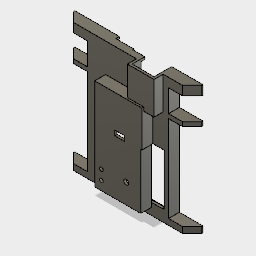
lpcCNC_Lid v15 (Autodesk Fusion 360 design; units mm, degrees)
Autodesk Fusion 360 part; units mm, degrees
sketch "Base Sketch" plane through (0, 0, 0) normal (0, 0, 1) x (1, 0, 0)
  line L0 (0, 0) -> (106, 0)
  line L1 (106, 0) -> (106, 106)
  line L2 (106, 106) -> (0, 106)
  line L3 (0, 106) -> (0, 0)
  line L4 (19.5, 106) -> (86.5, 106)
  line L5 (86.5, 106) -> (86.5, 0)
  line L6 (86.5, 0) -> (19.5, 0)
  line L7 (19.5, 0) -> (19.5, 106)
  line L8 (21.5, 3) -> (84.5, 3)
  line L9 (84.5, 3) -> (84.5, 104)
  line L10 (84.5, 104) -> (21.5, 104)
  line L11 (21.5, 104) -> (21.5, 3)
  circle A0 centre (23, 7) radius 3
  circle A1 centre (23, 7) radius 0.9
  circle A2 centre (83, 7) radius 0.9
  circle A3 centre (83, 7) radius 3
  circle A4 centre (83, 99) radius 0.9
  circle A5 centre (83, 99) radius 3
  circle A6 centre (23, 99) radius 0.9
  circle A7 centre (23, 99) radius 3
  line L12 (80, 106) -> (80, 104)
  line L13 (52, 106) -> (52, 104)
  line L14 (37, 106) -> (37, 104)
  line L15 (86.5, 5) -> (106, 5)
  line L16 (106, 5) -> (106, 0)
  line L17 (106, 0) -> (86.5, 0)
  line L18 (86.5, 0) -> (86.5, 5)
  line L19 (0, 5) -> (19.5, 5)
  line L20 (19.5, 5) -> (19.5, 0)
  line L21 (19.5, 0) -> (0, 0)
  line L22 (0, 0) -> (0, 5)
  line L23 (86.5, 106) -> (106, 106)
  line L24 (106, 106) -> (106, 98.5)
  line L25 (106, 98.5) -> (86.5, 98.5)
  line L26 (86.5, 98.5) -> (86.5, 106)
  line L27 (0, 106) -> (19.5, 106)
  line L28 (19.5, 106) -> (19.5, 98.5)
  line L29 (19.5, 98.5) -> (0, 98.5)
  line L30 (0, 98.5) -> (0, 106)
  line L31 (106, 76.5) -> (86.5, 76.5)
  line L32 (86.5, 76.5) -> (86.5, 80)
  line L33 (86.5, 80) -> (106, 80)
  line L34 (106, 80) -> (106, 76.5)
  line L35 (0, 76.5) -> (19.5, 76.5)
  line L36 (19.5, 76.5) -> (19.5, 80)
  line L37 (19.5, 80) -> (0, 80)
  line L38 (0, 80) -> (0, 76.5)
  line L39 (63.5, 104) -> (80, 104)
  line L40 (80, 104) -> (80, 81)
  line L41 (36.5, 8) -> (71.5, 8)
  line L42 (71.5, 52) -> (83, 52)
  line L43 (83, 52) -> (83, 9.5)
  line L44 (83, 9.5) -> (71.5, 9.5)
  line L45 (71.5, 9.5) -> (71.5, 52)
  line L46 (62, 106) -> (62, 104)
  line L47 (62, 104) -> (62, 81)
  line L48 (36.5, 80) -> (71.5, 80)
  line L49 (36.5, 80) -> (36.5, 8)
  line L50 (71.5, 8) -> (71.5, 80)
  line L51 (62, 81) -> (80, 81)
  line L52 (36.5, 80) -> (62, 80)
  line L53 (62, 80) -> (62, 82)
  line L54 (62, 82) -> (36.5, 82)
  line L55 (36.5, 82) -> (36.5, 80)
  line L56 (62, 106) -> (60, 106)
  line L57 (60, 106) -> (60, 82)
  line L58 (60, 82) -> (62, 82)
  line L59 (62, 82) -> (62, 106)
  line L60 (80, 81) -> (82, 81)
  line L61 (82, 81) -> (82, 106)
  line L62 (82, 106) -> (80, 106)
  line L63 (80, 106) -> (80, 81)
  line L64 (82, 81) -> (71.5, 81)
  line L65 (71.5, 81) -> (71.5, 79)
  line L66 (71.5, 79) -> (82, 79)
  line L67 (82, 79) -> (82, 81)
  line L68 (71.5, 79) -> (73.5, 79)
  line L69 (73.5, 79) -> (73.5, 52)
  line L70 (73.5, 52) -> (71.5, 52)
  line L71 (71.5, 52) -> (71.5, 79)
  line L72 (36.5, 82) -> (34.5, 82)
  line L73 (34.5, 82) -> (34.5, 6)
  line L74 (34.5, 6) -> (36.5, 6)
  line L75 (36.5, 6) -> (36.5, 82)
  line L76 (36.5, 6) -> (71.5, 6)
  line L77 (71.5, 6) -> (71.5, 8)
  line L78 (71.5, 8) -> (36.5, 8)
  line L79 (36.5, 8) -> (36.5, 6)
  line L80 (71.5, 6) -> (72.5, 6)
  line L81 (72.5, 6) -> (72.5, 52)
  line L82 (72.5, 52) -> (71.5, 52)
  line L83 (71.5, 52) -> (71.5, 6)
  line L84 (62, 81) -> (73.5, 81)
  line L85 (73.5, 81) -> (73.5, 82)
  line L86 (73.5, 82) -> (62, 82)
  line L87 (62, 82) -> (62, 81)
  line L88 (73.5, 81) -> (73.5, 79)
  line L89 (51, 55) -> (59, 55)
  line L90 (59, 55) -> (59, 51)
  line L91 (59, 51) -> (51, 51)
  line L92 (51, 51) -> (51, 55)
  circle A8 centre (60.5, 22.5) radius 2
  circle A9 centre (40, 21.5) radius 1.5
  circle A10 centre (40, 13.5) radius 1.5
  dimension "d1" = 106
  dimension "d2" = 106
  dimension "d4" = 67
  dimension "d5" = 19.5
  dimension "d6" = 63
  dimension "d8" = 2
  dimension "d9" = 3
  dimension "d10" = 6
  dimension "d12" = 6
  dimension "d13" = 6
  dimension "d14" = 6
  dimension "d15" = 23
  dimension "d16" = 23
  dimension "d17" = 23
  dimension "d18" = 23
  dimension "d19" = 7
  dimension "d20" = 7
  dimension "d21" = 7
  dimension "d22" = 7
  dimension "d24" = 2
  dimension "d25" = 6.5
  dimension "d28" = 15
  dimension "d35" = 5
  dimension "d36" = 5
  dimension "d37" = 7.5
  dimension "d38" = 7.5
  dimension "d39" = 3.5
  dimension "d40" = 26
  dimension "d41" = 3.5
  dimension "d42" = 26
  dimension "d45" = 8
  dimension "d48" = 42.5
  dimension "d49" = 9.5
  dimension "d60" = 10
  dimension "d62" = 18
  dimension "d63" = 1.8
  dimension "d64" = 1.8
  dimension "d65" = 1.8
  dimension "d66" = 1.8
  dimension "d68" = 72
  dimension "d69" = 25
  dimension "d70" = 35
  dimension "d71" = 2
  dimension "d72" = 2
  dimension "d73" = 2
  dimension "d74" = 2
  dimension "d75" = 2
  dimension "d76" = 11.5
  dimension "d77" = 2
  dimension "d78" = 2
  dimension "d87" = 1
  dimension "d88" = 25.5
  dimension "d89" = 44
  dimension "d90" = 36.5
  dimension "d94" = 1
  dimension "d95" = 11.5
  dimension "d96" = 8
  dimension "d97" = 4
  dimension "d98" = 25
  dimension "d99" = 14.5
  dimension "d100" = 4
  dimension "d101" = 3
  dimension "d102" = 3
  dimension "d103" = 5.5
  dimension "d104" = 13.5
  dimension "d105" = 3.5
  dimension "d106" = 3.5
  dimension "d107" = 14.5
  dimension "d108" = 24
  measures "d1" distance of L0.start L0.end
  measures "d2" distance of L0.start L2.end
  measures "d4" distance of L4.start L4.end
  measures "d5" distance of L3 L7
  measures "d6" distance of L8.start L8.end
  measures "d8" distance of L7 L11
  measures "d9" distance of L0 L8
  measures "d10" diameter of A0
  measures "d12" diameter of A3
  measures "d13" diameter of A5
  measures "d14" diameter of A7
  measures "d15" distance of L3 A0.centre
  measures "d16" distance of L1 A2.centre
  measures "d17" distance of L3 A6.centre
  measures "d18" distance of L1 A4.centre
  measures "d19" distance of L4 A6.centre
  measures "d20" distance of L2 A4.centre
  measures "d21" distance of L0 A2.centre
  measures "d22" distance of L0 A0.centre
  measures "d24" distance of L2 L10
  measures "d25" distance of L5 L12
  measures "d28" distance of L13 L14
  measures "d35" distance of L0 L19
  measures "d36" distance of L15 L17
  measures "d37" distance of L27 L29
  measures "d38" distance of L2 L25
  measures "d39" distance of L31 L33
  measures "d40" distance of L2 L33
  measures "d41" distance of L35 L37
  measures "d42" distance of L2 L37
  measures "d45" distance of L0 L41
  measures "d48" distance of L42 L44
  measures "d49" distance of L0 L44
  measures "d60" distance of L13 L46
  measures "d62" distance of L40 L47
  measures "d63" diameter of A6
  measures "d64" diameter of A4
  measures "d65" diameter of A1
  measures "d66" diameter of A2
  measures "d68" distance of L41 L48
  measures "d69" distance of L4 L51
  measures "d70" distance of L49 L50
  measures "d71" distance of L48 L54
  measures "d72" distance of L47 L57
  measures "d73" distance of L61 L63
  measures "d74" distance of L51 L66
  measures "d75" distance of L50 L69
  measures "d76" distance of L43 L45
  measures "d77" distance of L49 L73
  measures "d78" distance of L76 L78
  measures "d87" distance of L45 L81
  measures "d88" distance of L53 L75
  measures "d89" distance of L1 L59
  measures "d90" distance of L3 L49
  measures "d94" distance of L84 L86
  measures "d95" distance of L53.end L85
  measures "d96" distance of L89.start L89.end
  measures "d97" distance of L89.start L91.end
  measures "d98" distance of L52 L89
  measures "d99" distance of L49 L92
  measures "d100" diameter of A8
  measures "d101" diameter of A9
  measures "d102" diameter of A10
  measures "d103" distance of L78 A10.centre
  measures "d104" distance of L41 A9.centre
  measures "d105" distance of L49 A9.centre
  measures "d106" distance of L49 A10.centre
  measures "d107" distance of L78 A8.centre
  measures "d108" distance of L49 A8.centre
extrude "Extrude1" add sketch "Base Sketch" against normal blind 9 contours L0 L3 L7 L19 L20 L21 L22 | L0 L2 L4 L5 L6 L7 L8 L9 L10 L11 A0 A3 A5 A7 L14 L18 L20 L26 L28 L32 L36 L61 | L0 L1 L5 L15 L16 L17 L18 | L3 L7 L35 L36 L37 L38 | L1 L5 L31 L32 L33 L34 | L2 L3 L7 L27 L28 L29 L30 | L1 L2 L5 L23 L24 L25 L26 | L2 L4 L10 L12 L61 L62 L63 | A5 L61 | L9 A5 L61 | L11 A7 | L11 A7 | L9 A5 | L11 A0 | L11 A0 | L9 A3 | L9 A3 L43 L44 | A3 L43 L44 makes body 1
extrude "Extrude2" add sketch "Base Sketch" against normal blind 6 contours L2 L4 L10 L13 L14 bodies 1
extrude "Extrude3" add sketch "Base Sketch" against normal blind 5 contours L2 L4 L10 L13 L57 | L2 L4 L10 L46 L56 L57 L59 bodies 1
extrude "Extrude4" add sketch "Base Sketch" against normal blind 2 separate body contours L0 L2 L4 L5 L6 L7 L8 L9 L10 L11 A0 A3 A5 A7 L14 L18 L20 L26 L28 L32 L36 L61 | L2 L4 L10 L13 L14 | L2 L4 L10 L12 L61 L62 L63 | L2 L4 L10 L13 L57 | L8 L9 L10 L11 A0 A3 A7 L44 L54 L57 L72 L73 L74 L76 L80 L81 | L10 A5 L40 L61 L63 | L9 L10 A5 L61 | L2 L4 L10 L46 L56 L57 L59 | A5 L61 | L9 A5 L61 | L10 L47 L54 L57 L58 L59 | L11 A7 | L11 A7 | A5 L40 L60 L61 L63 L64 | L9 A5 | L9 A3 A5 L42 L43 L61 L66 L67 L69 | L47 L48 L52 L53 L54 L55 L58 L75 L87 | L51 L60 L64 L66 L67 L88 | L49 L55 L72 L73 L74 L75 L79 | L11 A0 | L11 A0 | L48 L51 L53 L65 L84 | L50 L51 L64 L65 L66 L68 L84 L88 | L9 A3 | L9 A3 L43 L44 | L42 L50 L66 L68 L69 L70 L71 L82 | A3 L43 L44 | L41 L75 L76 L77 L78 L79 L83 | L44 L50 L77 L80 L81 L83 | A1 | A2 | A4 | A6 makes body 2
chamfer "Chamfer1" distance 8 angle 45 1 edges at (106, 102.25, 0) on bodies 1
chamfer "Chamfer2" distance 8 angle 45 1 edges at (106, 78.25, 0) on bodies 1
chamfer "Chamfer3" distance 8 angle 45 1 edges at (106, 2.5, 0) on bodies 1
chamfer "Chamfer4" distance 8 angle 45 1 edges at (0, 102.25, 0) on bodies 1
chamfer "Chamfer5" distance 8 angle 45 1 edges at (0, 78.25, 0) on bodies 1
chamfer "Chamfer6" distance 8 angle 45 1 edges at (0, 2.5, 0) on bodies 1
extrude "Extrude5" add sketch "Base Sketch" along normal blind 7 contours L47 L48 L52 L53 L54 L55 L58 L75 L87 | L49 L55 L72 L73 L74 L75 L79 | L48 L51 L53 L65 L84 | L50 L51 L64 L65 L66 L68 L84 L88 | L42 L50 L66 L68 L69 L70 L71 L82 | L41 L75 L76 L77 L78 L79 L83 | L44 L50 L77 L80 L81 L83 | L42 L44 L45 L50 L70 L81 L82 L83 bodies 2
extrude "Extrude6" add sketch "Base Sketch" along normal blind 2 from surface at 7 separate body contours L47 L48 L52 L53 L54 L55 L58 L75 L87 | L49 L55 L72 L73 L74 L75 L79 | L48 L51 L53 L65 L84 | L50 L51 L64 L65 L66 L68 L84 L88 | L41 L45 L48 L49 L50 L52 L65 L71 L75 L78 L83 | L42 L50 L66 L68 L69 L70 L71 L82 | L41 L75 L76 L77 L78 L79 L83 | L44 L50 L77 L80 L81 L83 | L42 L44 L45 L50 L70 L81 L82 L83 makes body 3
extrude "Extrude7" add sketch "Base Sketch" along normal blind 5.5 contours L2 L4 L10 L12 L61 L62 L63 | L10 A5 L40 L61 L63 | L2 L4 L10 L46 L56 L57 L59 | A5 L61 | L10 L47 L54 L57 L58 L59 | A5 L40 L60 L61 L63 L64 | L51 L60 L64 L66 L67 L88 bodies 2 1
extrude "Extrude8" add sketch "Base Sketch" along normal blind 2 from surface at 5.5 separate body contours L2 L4 L10 L12 L61 L62 L63 | L2 L4 L10 L12 L39 L46 L59 L63 | L10 A5 L40 L61 L63 | L2 L4 L10 L46 L56 L57 L59 | L10 L39 L40 L47 L51 L59 L63 L64 L85 L86 | A5 L61 | L10 L47 L54 L57 L58 L59 | A5 L40 L60 L61 L63 L64 | L51 L60 L64 L66 L67 L88 makes body 4
extrude "Extrude9" add sketch "Base Sketch" along normal blind 3.5 from surface at 5.5 contours L47 L51 L53 L64 L84 L85 L86 L87 bodies 2 3 4
